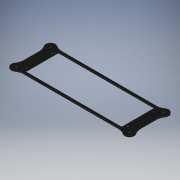
# Autodesk Inventor part: Base2
Saved by Autodesk Inventor 2017 (Build 210142000, 142)
## iProperties
Created: 2017-04-15
Part Number: Base2
Material: Generic
Document SubType Name: Modeling
Designer: jeffkub
Density: 1 g/cm^3
Appearance: Default(2)
Author: jeffkub
Autodesk Inventor part; units mm, degrees
ref_plane "YZ Plane" through (0, 0, 0) normal (1, 0, 0) x (0, 1, 0)
ref_plane "XZ Plane" through (0, 0, 0) normal (0, 1, 0) x (-1, 0, 0)
ref_plane "XY Plane" through (0, 0, 0) normal (0, 0, 1) x (1, 0, 0)
sketch "Sketch2" plane through (0, 0, 0) normal (0, 1, 0) x (-1, 0, 0)
  line L0 (-94, 28.5) -> (94, 28.5) construction
  line L1 (94, 28.5) -> (94, -28.5) construction
  line L2 (94, -28.5) -> (-94, -28.5) construction
  line L3 (-94, -28.5) -> (-94, 28.5) construction
  line L4 (-94, 28.5) -> (94, -28.5) construction
  line L5 (94, 28.5) -> (-94, -28.5) construction
  line L6 (78.6703, -31.5) -> (-78.6703, -31.5)
  line L7 (-97, -13.1703) -> (-97, 13.1703)
  line L8 (-78.6703, 31.5) -> (78.6703, 31.5)
  line L9 (97, 13.1703) -> (97, -13.1703)
  arc A0 (89.2832, -34.9615) -> (100.4615, -23.7832) centre (94, -28.5) ccw
  arc A1 (100.4615, 23.7832) -> (89.2832, 34.9615) centre (94, 28.5) ccw
  arc A2 (-89.2832, 34.9615) -> (-100.4615, 23.7832) centre (-94, 28.5) ccw
  arc A3 (-100.4615, -23.7832) -> (-89.2832, -34.9615) centre (-94, -28.5) ccw
  arc A4 (89.2832, -34.9615) -> (78.6703, -31.5) centre (78.6703, -49.5) ccw
  arc A5 (97, -13.1703) -> (100.4615, -23.7832) centre (115, -13.1703) ccw
  arc A6 (100.4615, 23.7832) -> (97, 13.1703) centre (115, 13.1703) ccw
  arc A7 (78.6703, 31.5) -> (89.2832, 34.9615) centre (78.6703, 49.5) ccw
  arc A8 (-89.2832, 34.9615) -> (-78.6703, 31.5) centre (-78.6703, 49.5) ccw
  arc A9 (-97, 13.1703) -> (-100.4615, 23.7832) centre (-115, 13.1703) ccw
  arc A10 (-100.4615, -23.7832) -> (-97, -13.1703) centre (-115, -13.1703) ccw
  arc A11 (-78.6703, -31.5) -> (-89.2832, -34.9615) centre (-78.6703, -49.5) ccw
  circle A12 centre (94, -28.5) radius 1.6
  circle A13 centre (94, 28.5) radius 1.6
  circle A14 centre (-94, -28.5) radius 1.6
  circle A15 centre (-94, 28.5) radius 1.6
  circle A16 centre (94, -28.5) radius 3 construction
  circle A17 centre (94, 28.5) radius 3 construction
  circle A18 centre (-94, 28.5) radius 3 construction
  circle A19 centre (-94, -28.5) radius 3 construction
  point P0 (0, 0)
  point P1 (86.5838, -31.5)
  point P2 (-86.5838, -31.5)
  point P3 (-97, -21.0838)
  point P4 (-97, 21.0838)
  point P5 (-86.5838, 31.5)
  point P6 (86.5838, 31.5)
  point P7 (97, 21.0838)
  point P8 (97, -21.0838)
  dimension "d6" = 3
  dimension "d7" = 3
  dimension "d8" = 3
  dimension "d9" = 3
  dimension "d10" = 8
  dimension "d11" = 18
  dimension "d14" = 3.2
  dimension "d15" = 63
  dimension "d16" = 194
  dimension "d17" = 6
  constraints: 32 point on circle, 20 centre point, 20 end point, 16 equal radius, 16 tangent, 12 coincident, 8 point on line, 3 horizontal, 3 parallel, 2 midpoint, 1 perpendicular, 1 vertical
  measures "d6" distance between parallel lines of L2 L6
  measures "d7" distance between parallel lines of L8 L0
  measures "d8" distance between parallel lines of L1 L9
  measures "d9" distance between parallel lines of L3 L7
  measures "d10" radius of A0
  measures "d11" radius of A4
  measures "d14" diameter of A12
  measures "d15" distance between parallel lines of L8 L6
  measures "d16" distance between parallel lines of L7 L9
  measures "d17" diameter of A16
extrude "Extrusion1" add sketch "Sketch2" along normal blind 1.5
sketch "Sketch3" plane through (0, 1.5, 0) normal (0, 1, 0) x (1, 0, 0)
  line L0 (84, -21) -> (-84, -21) construction
  line L1 (-84, -21) -> (-84, 21) construction
  line L2 (-84, 21) -> (84, 21) construction
  line L3 (84, 21) -> (84, -21) construction
  line L4 (84, -21) -> (-84, 21) construction
  line L5 (-84, -21) -> (84, 21) construction
  circle A0 centre (-84, 21) radius 1.6
  circle A1 centre (-84, -21) radius 1.6
  circle A2 centre (84, -21) radius 1.6
  circle A3 centre (84, 21) radius 1.6
  line L6 (-78, 27.5) -> (78, 27.5)
  line L7 (80, 25.5) -> (80, -25.5)
  line L8 (78, -27.5) -> (-78, -27.5)
  line L9 (-80, -25.5) -> (-80, 25.5)
  arc A4 (-78, 27.5) -> (-80, 25.5) centre (-78, 25.5) ccw
  arc A5 (-80, -25.5) -> (-78, -27.5) centre (-78, -25.5) ccw
  arc A6 (78, -27.5) -> (80, -25.5) centre (78, -25.5) ccw
  arc A7 (80, 25.5) -> (78, 27.5) centre (78, 25.5) ccw
  point P0 (0, 0)
  point P1 (-80, 0)
  point P2 (0, 0)
  point P3 (0, 27.5)
  point P4 (0, 0)
  dimension "d18" = 168
  dimension "d19" = 42
  dimension "d20" = 3.2
  dimension "d23" = 2
  dimension "d24" = 160
  dimension "d25" = 55
  constraints: 20 end point, 8 centre point, 8 point on circle, 8 tangent, 6 equal radius, 6 midpoint, 4 coincident, 4 parallel, 2 horizontal, 2 perpendicular, 1 horizontal alignment, 1 vertical alignment
  measures "d18" distance of L1.end L2.end
  measures "d19" distance of L2.end L0.start
  measures "d20" diameter of A0
  measures "d23" radius of A4
  measures "d24" distance between parallel lines of L7 L9
  measures "d25" distance between parallel lines of L8 L6
extrude "Extrusion2" cut sketch "Sketch3" against normal through all
equation "\"d7\" = d6"
equation "\"d8\" = d6"
equation "\"d9\" = d8"
equation "\"d21\" = d20"
body "Solid1"
